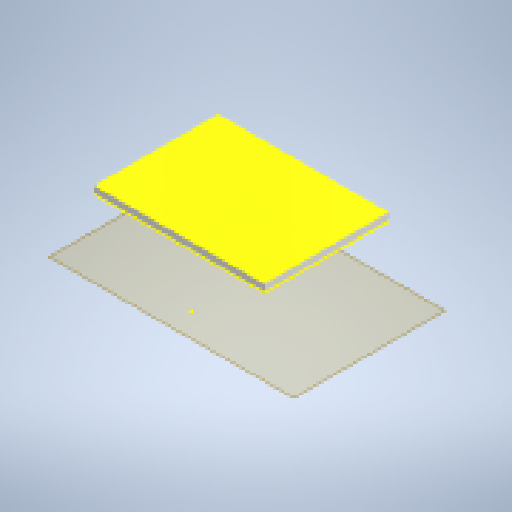
# Autodesk Inventor part: Sleed_Plate
Saved by Autodesk Inventor 2024 (Build 280153000, 153)
## iProperties
Created: 2023-11-25
Part Number: Sleed_Plate
Material: Generic
Document SubType Name: Modeling
Designer: danie
Density: 1 g/cm^3
Appearance: Default
Author: danie
Autodesk Inventor part; units mm, degrees
ref_plane "YZ Plane" through (0, 0, 0) normal (1, 0, 0) x (0, 1, 0)
ref_plane "XZ Plane" through (0, 0, 0) normal (0, 1, 0) x (-1, 0, 0)
ref_plane "XY Plane" through (0, 0, 0) normal (0, 0, 1) x (1, 0, 0)
ref_plane "Work Plane2" through (-92.9211, 111.7581, -85.645) normal (0, 1, 0) x (-1, 0, 0)
sketch "Sketch2" plane through (-92.9211, 111.7581, -85.645) normal (0, 1, 0) x (-1, 0, 0)
  line L0 (63, 0) -> (-63, 0)
  line L1 (-63, 0) -> (-63, -150)
  line L2 (-63, -150) -> (63, -150)
  line L3 (63, -150) -> (63, 0)
  line L4 (63, 0) -> (-63, -150) construction
  line L5 (-63, 0) -> (63, -150) construction
  line L6 (-114.9576, 160) -> (114.9576, 160)
  line L7 (114.9576, 160) -> (114.9576, -160)
  line L8 (114.9576, -160) -> (-114.9576, -160)
  line L9 (-114.9576, -160) -> (-114.9576, 160)
  line L10 (119.9576, -165) -> (119.9576, 165)
  line L11 (119.9576, 165) -> (-119.9576, 165)
  line L12 (-119.9576, 165) -> (-119.9576, 10)
  line L13 (-119.9576, -165) -> (119.9576, -165)
  line L14 (-119.9576, 10) -> (-114.9576, 10)
  line L15 (-114.9576, 10) -> (114.9576, 10)
  line L16 (114.9576, 10) -> (119.9576, 10)
  line L17 (-119.9576, 10) -> (-119.9576, -165)
  point P0 (-92.9211, 85.645)
  point P1 (0, -75)
  point P2 (114.9576, 160)
  dimension "d0" = 126
  dimension "d1" = 150
  dimension "d2" = 5
  dimension "d5" = 10
  dimension "d6" = 10
  constraints: 36 end point, 7 parallel, 6 perpendicular, 3 point on line, 2 horizontal, 2 midpoint, 4 other
  measures "d0" distance of L2.end L1.end
  measures "d1" distance of L1.end L0.end
  measures "d2" distance between parallel lines of L7 L10
  measures "d5" distance between parallel lines of L8 L2
  measures "d6" distance between parallel lines of L14 L0
extrude "Extrusion1" add sketch "Sketch2" along normal blind 10 contours L3 L2 L1 L0 | L15 L7 L8 L9 | L9 L8 L7 L16 L10 L13 L17 L14
sketch "Sketch3" plane through (-92.9211, 111.7581, -85.645) normal (0, -1, 0) x (1, 0, 0)
  line L0 (-119.9576, 10) -> (119.9576, 10) projected
  line L1 (-119.9576, -165) -> (-119.9576, 10) projected
  line L2 (119.9576, -165) -> (-119.9576, -165) projected
  line L3 (119.9576, 10) -> (119.9576, -165) projected
  line L4 (-119.9576, -165) -> (119.9576, 10)
  line L5 (-119.9576, 10) -> (119.9576, -165)
  circle A0 centre (0, -77.5) radius 37.5
  point P0 (92.9211, 85.645)
  dimension "d7" = 75
  constraints: 4 end point, 1 centre point, 1 midpoint
  measures "d7" diameter of A0
extrude "Extrusion2" cut sketch "Sketch3" against normal through all contours A0 L4 L5 | L5 L4 A0 | A0 L5 L4 | L4 L5 A0
sketch "Sketch4" plane through (-92.9211, 111.7581, -85.645) normal (0, -1, 0) x (1, 0, 0)
  circle A0 centre (-37.5, -38.6758) radius 2.5 projected
  circle A1 centre (37.5, -38.6758) radius 2.5 projected
  circle A2 centre (37.5, -116.3242) radius 2.5 projected
  circle A3 centre (-37.5, -116.3242) radius 2.5 projected
  arc A4 (47.5, -35) -> (42.5, -30) centre (42.5, -35) ccw projected
  line L0 (42.5, -30) -> (-42.5, -30) projected
  arc A5 (-42.5, -30) -> (-47.5, -35) centre (-42.5, -35) ccw projected
  line L1 (-47.5, -35) -> (-47.5, -120) projected
  arc A6 (-47.5, -120) -> (-42.5, -125) centre (-42.5, -120) ccw projected
  line L2 (-42.5, -125) -> (42.5, -125) projected
  arc A7 (42.5, -125) -> (47.5, -120) centre (42.5, -120) ccw projected
  line L3 (47.5, -120) -> (47.5, -35) projected
  circle A8 centre (0, -77.5) radius 5 projected
  point P0 (92.9211, 85.645)
hole "Hole1" at (-130.4211, 111.7581, -124.3208) at (-55.4211, 111.7581, -124.3208) at (-55.4211, 111.7581, -201.9692) at (-130.4211, 111.7581, -201.9692) direction (0, 1, 0) diameter 5 end through all
body "Solid1"
